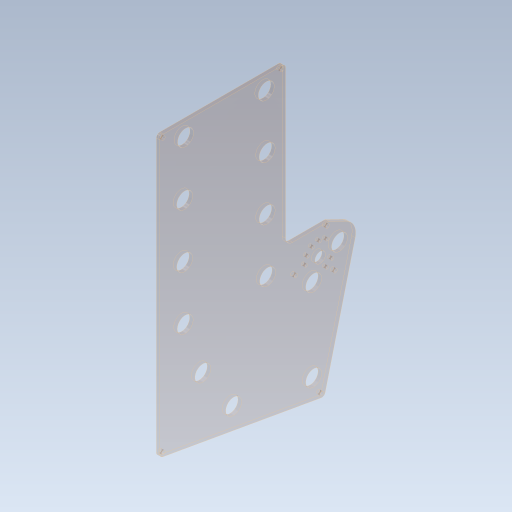
# Autodesk Inventor part: sketchers
Saved by Autodesk Inventor 2024 (Build 280153000, 153)
## iProperties
Created: 2024-07-27
Part Number: sketchers
Material: Polycarbonate, Smoke
Document SubType Name: Modeling
Designer: Oscar
Density: 1.2 g/cm^3
Appearance: Polycarbonate - Smoked
Author: Oscar
Autodesk Inventor part; units mm, degrees
ref_plane "YZ Plane" through (0, 0, 0) normal (1, 0, 0) x (0, 1, 0)
ref_plane "XZ Plane" through (0, 0, 0) normal (0, 1, 0) x (-1, 0, 0)
ref_plane "XY Plane" through (0, 0, 0) normal (0, 0, 1) x (1, 0, 0)
sketch "Sketch1" plane through (0, 0, 0) normal (1, 0, 0) x (0, 1, 0)
  line L0 (95.25, 812.8) -> (44.45, 812.8) construction
  line L1 (44.45, 812.8) -> (44.45, 0) construction
  line L2 (44.45, 0) -> (95.25, 0) construction
  line L3 (95.25, 0) -> (95.25, 812.8) construction
  line L4 (95.25, 0) -> (44.45, 0) construction
  line L5 (44.45, 0) -> (44.45, 25.4) construction
  line L6 (44.45, 25.4) -> (95.25, 25.4) construction
  line L7 (95.25, 25.4) -> (95.25, 0) construction
  circle A0 centre (190.5, 0) radius 50.8 construction
  circle A1 centre (95.25, 279.4) radius 25.4 construction
  circle A2 centre (278.0133, 267.5807) radius 9.525
  circle A3 centre (278.0133, 267.5807) radius 25.4 construction
  circle A4 centre (278.0133, 267.5807) radius 31.75 construction
  circle A5 centre (303.4133, 267.5807) radius 2.4892
  circle A6 centre (300.0104, 280.2807) radius 2.4892
  circle A7 centre (290.7133, 289.5778) radius 2.4892
  circle A8 centre (278.0133, 292.9807) radius 2.4892
  circle A9 centre (265.3133, 289.5778) radius 2.4892 construction
  circle A10 centre (256.0163, 280.2807) radius 2.4892 construction
  circle A11 centre (252.6133, 267.5807) radius 2.4892 construction
  circle A12 centre (256.0163, 254.8807) radius 2.4892
  circle A13 centre (265.3133, 245.5837) radius 2.4892
  circle A14 centre (278.0133, 242.1807) radius 2.4892 construction
  circle A15 centre (290.7133, 245.5837) radius 2.4892 construction
  circle A16 centre (300.0104, 254.8807) radius 2.4892
  circle A17 centre (609.6, 438.15) radius 50.8 construction
  circle A18 centre (278.0133, 267.5807) radius 30.48 construction
  circle A19 centre (587.8333, 365.125) radius 25.4 construction
  circle A20 centre (587.8333, 511.175) radius 25.4 construction
  line L8 (587.8333, 485.775) -> (587.8333, 390.525) construction
  circle A21 centre (490.3356, 512.7625) radius 14.351
  circle A22 centre (392.825, 512.7625) radius 14.351
  circle A23 centre (490.3356, 363.5375) radius 14.351
  line L9 (587.8333, 511.175) -> (490.3356, 512.7625) construction
  line L10 (587.8333, 365.125) -> (490.3356, 363.5375) construction
  circle A24 centre (490.3356, 512.7625) radius 25.4 construction
  circle A25 centre (490.3356, 363.5375) radius 25.4 construction
  line L11 (490.3356, 487.3625) -> (490.3356, 388.9375) construction
  circle A26 centre (392.825, 512.7625) radius 25.4 construction
  circle A27 centre (392.825, 363.5375) radius 25.4 construction
  circle A28 centre (392.825, 363.5375) radius 14.351
  line L12 (490.3356, 512.7625) -> (392.825, 512.7625) construction
  line L13 (490.3356, 363.5375) -> (392.825, 363.5375) construction
  line L14 (392.825, 487.3625) -> (392.825, 388.9375) construction
  circle A29 centre (295.3189, 511.8309) radius 25.4 construction
  circle A30 centre (295.3189, 362.6059) radius 25.4 construction
  circle A31 centre (203.1597, 479.9719) radius 25.4 construction
  circle A32 centre (295.3189, 511.8309) radius 14.351
  circle A33 centre (295.3189, 362.6059) radius 14.351
  circle A34 centre (203.1597, 479.9719) radius 14.351
  line L15 (392.825, 512.7625) -> (295.3189, 511.8309) construction
  line L16 (392.825, 363.5375) -> (295.3189, 362.6059) construction
  line L17 (295.3189, 486.4309) -> (295.3189, 388.0059) construction
  line L18 (295.3189, 511.8309) -> (203.1597, 479.9719) construction
  circle A35 centre (123.1487, 424.2353) radius 25.4 construction
  circle A36 centre (123.1487, 424.2353) radius 14.351
  line L19 (203.1597, 479.9719) -> (123.1487, 424.2353) construction
  circle A37 centre (95.25, 279.4) radius 14.351
  circle A38 centre (407.176, 125.0684) radius 50.8 construction
  line L20 (609.6, 355.6) -> (44.45, 355.6) construction
  line L21 (44.45, 355.6) -> (44.45, 330.2) construction
  line L22 (44.45, 330.2) -> (609.6, 330.2) construction
  line L23 (609.6, 330.2) -> (609.6, 355.6) construction
  line L24 (95.25, 241.3) -> (44.45, 241.3) construction
  line L25 (44.45, 241.3) -> (44.45, 215.9) construction
  line L26 (44.45, 215.9) -> (95.25, 215.9) construction
  line L27 (95.25, 215.9) -> (95.25, 241.3) construction
  circle A39 centre (244.475, 279.4) radius 25.4 construction
  circle A40 centre (244.475, 279.4) radius 14.351
  line L28 (218.8463, 459.9947) -> (279.6322, 382.5831) construction
  circle A41 centre (278.0133, 267.5807) radius 8.89 construction
  circle A42 centre (284.5531, 232.6273) radius 26.67 construction
  circle A43 centre (244.475, 279.4) radius 26.67 construction
  circle A44 centre (284.5531, 232.6273) radius 14.351
  circle A45 centre (587.8333, 511.175) radius 14.351
  circle A46 centre (587.8333, 365.125) radius 14.351
  line L29 (44.45, 623.1841) -> (44.45, 648.5841) construction
  line L30 (95.25, 647.7) -> (609.6, 647.7) construction
  line L31 (609.6, 647.7) -> (609.6, 622.3) construction
  line L32 (609.6, 622.3) -> (95.25, 622.3) construction
  line L33 (95.25, 622.3) -> (95.25, 647.7) construction
  circle A47 centre (606.8833, 551.3359) radius 3.2639
  circle A48 centre (606.8833, 551.3359) radius 6.35 construction
  circle A49 centre (606.8833, 336.55) radius 3.2639
  circle A50 centre (606.8833, 336.55) radius 6.35 construction
  circle A51 centre (114.3, 551.3359) radius 3.2639
  circle A52 centre (114.3, 551.3359) radius 6.35 construction
  line L34 (598.719, 534.1241) -> (604.1619, 545.5987) construction
  line L35 (613.2333, 551.3359) -> (613.2333, 511.175)
  line L36 (613.2333, 365.125) -> (613.2333, 336.55)
  line L37 (613.2333, 511.175) -> (613.2333, 365.125)
  circle A53 centre (63.5, 264.8503) radius 3.2639
  circle A54 centre (63.5, 264.8503) radius 6.35 construction
  line L38 (339.48, 330.2) -> (606.8833, 330.2)
  line L39 (313.4556, 344.8233) -> (322.5239, 335.932) construction
  circle A55 centre (284.5531, 232.6273) radius 29.21 construction
  circle A56 centre (244.475, 279.4) radius 29.21 construction
  arc A57 (606.8833, 330.2) -> (613.2333, 336.55) centre (606.8833, 336.55) ccw
  line L40 (72.1591, 268.8184) -> (69.2727, 267.4957) construction
  line L41 (609.6, 342.9) -> (44.45, 342.9) construction
  circle A58 centre (284.5531, 232.6273) radius 19.05 construction
  line L42 (263.4811, 257.2191) -> (265.547, 254.8082) construction
  circle A59 centre (320.43, 254.2906) radius 3.2639
  circle A60 centre (271.3806, 311.5331) radius 3.2639
  circle A61 centre (243.2709, 239.8541) radius 3.2639
  line L43 (95.25, 558.8) -> (44.45, 558.8) construction
  line L44 (44.45, 558.8) -> (44.45, 533.4) construction
  line L45 (44.45, 533.4) -> (95.25, 533.4) construction
  line L46 (95.25, 533.4) -> (95.25, 558.8) construction
  line L47 (114.3, 557.6859) -> (606.8833, 557.6859)
  line L48 (108.0475, 552.4446) -> (57.2475, 265.959)
  line L49 (277.4039, 204.3057) -> (61.9458, 258.6935)
  circle A62 centre (320.43, 254.2906) radius 6.35 construction
  circle A63 centre (271.3806, 311.5331) radius 6.35 construction
  circle A64 centre (243.2709, 239.8541) radius 6.35 construction
  arc A65 (114.3, 557.6859) -> (108.0475, 552.4446) centre (114.3, 551.3359) ccw
  arc A66 (57.2475, 265.959) -> (61.9458, 258.6935) centre (63.5, 264.8503) ccw
  line L50 (314.3705, 256.1892) -> (308.3109, 258.0878) construction
  line L51 (314.9941, 251.0083) -> (309.5582, 247.7259) construction
  line L52 (272.3281, 305.2542) -> (273.2757, 298.9753) construction
  line L53 (267.304, 306.6644) -> (263.2274, 301.7958) construction
  line L54 (249.5258, 238.7591) -> (255.7807, 237.6641) construction
  line L55 (248.2341, 243.815) -> (253.1973, 247.776) construction
  line L56 (326.78, 317.5) -> (326.78, 254.2906)
  arc A67 (339.48, 330.2) -> (326.78, 317.5) centre (339.48, 317.5) ccw
  line L57 (326.1461, 251.5249) -> (310.8471, 219.9051)
  arc A68 (326.1461, 251.5249) -> (326.78, 254.2906) centre (320.43, 254.2906) ccw
  arc A69 (277.4039, 204.3057) -> (310.8471, 219.9051) centre (284.5531, 232.6273) ccw
  arc A70 (613.2333, 551.3359) -> (606.8833, 557.6859) centre (606.8833, 551.3359) ccw
  point P0 (0, 0)
  point P1 (273.7117, 242.0302)
  point P2 (272.9427, 241.0623)
  point P3 (254.5339, 269.1643)
  point P4 (250.4488, 266.3515)
  dimension "d9" = 50.8
  dimension "d14" = 50.8
  dimension "d53" = 50.8
  dimension "d1" = 812.8
  dimension "d2" = 44.45
  dimension "d4" = 25.4
  dimension "d5" = 101.6
  dimension "d6" = 95.25
  dimension "d8" = 50.8
  dimension "d15" = 63.5
  dimension "d21" = 19.05
  dimension "d26" = 360
  dimension "d28" = 4.9784
  dimension "d29" = 438.15
  dimension "d30" = 514.35
  dimension "d36" = 60.96
  dimension "d38" = 50.8
  dimension "d39" = 50.8
  dimension "d41" = 95.25
  dimension "d45" = 28.702
  dimension "d47" = 97.5106
  dimension "d48" = 98.425
  dimension "d56" = 25.4
  dimension "d73" = 50.8
  dimension "d74" = 25.4
  dimension "d75" = 215.9
  dimension "d78" = 279.4
  dimension "d80" = 149.225
  dimension "d81" = 97.5106
  dimension "d82" = 147.4978
  dimension "d83" = 17.78
  dimension "d85" = 53.34
  dimension "d92" = 330.2
  dimension "d100" = 514.35
  dimension "d107" = 25.4
  dimension "d108" = 514.35
  dimension "d109" = 266.7
  dimension "d110" = 12.7
  dimension "d115" = 6.5278
  dimension "d116" = 12.7
  dimension "d122" = 2.54
  dimension "d123" = 2.54
  dimension "d128" = 3.175
  dimension "d133" = 38.1
  dimension "d134" = 3.175
  dimension "d135" = 194.9958
  dimension "d136" = 6.5278
  dimension "d137" = 25.4
  dimension "d138" = 533.4
  dimension "d139" = 19.05
  dimension "d140" = 19.05
  dimension "d141" = 12.7
  dimension "d142" = 6.35
  dimension "d143" = 12.7
  constraints: 114 end point, 63 centre point, 51 point on circle, 32 point on line, 27 coincident, 25 tangent, 24 equal radius, 15 equal length, 11 parallel, 9 horizontal, 7 vertical alignment, 6 horizontal alignment, 6 perpendicular, 4 concentric, 4 vertical, 2 midpoint, 53 other
  measures "d1" distance of L1.end L0.end
  measures "d2" distance from line of point (0, 0) L1
  measures "d4" distance of L4.end L5.end
  measures "d5" diameter of A0
  measures "d15" diameter of A4
  measures "d21" diameter of A2
  measures "d28" diameter of A16
  measures "d29" distance from line of L2 point (609.6, 438.15)
  measures "d36" diameter of A18
  measures "d38" diameter of A19
  measures "d39" diameter of A20
  measures "d41" distance of L8.start L8.end
  measures "d45" diameter of A21
  measures "d47" distance of L9.start L9.end
  measures "d48" distance of L11.start L11.end
  measures "d56" distance of L22.end L20.start
  measures "d73" distance of L26.end L25.end
  measures "d74" distance of L25.end L24.end
  measures "d75" distance between parallel lines of L2 L26
  measures "d78" distance from line of L2 point (95.25, 279.4)
  measures "d80" distance of point (95.25, 279.4) A39.centre
  measures "d81" distance of A39.centre A30.centre
  measures "d82" distance of point (95.25, 279.4) A35.centre
  measures "d83" diameter of A41
  measures "d85" diameter of A42
  measures "d92" distance between parallel lines of L2 L22
  measures "d107" distance between parallel lines of L32 L30
  measures "d108" distance of L31.end L32.end
  measures "d109" distance between parallel lines of L20 L32
  measures "d110" distance of L34.start L34.end
  measures "d115" diameter of A47
  measures "d116" diameter of A48
  measures "d122" radial gap between concentric circles of A42 A55
  measures "d123" radial gap between concentric circles of A43 A56
  measures "d128" distance of L40.start L40.end
  measures "d133" diameter of A58
  measures "d134" distance of L42.start L42.end
  measures "d135" distance of A37.centre A44.centre
  measures "d136" diameter of A61
  measures "d137" distance between parallel lines of L43 L45
  measures "d138" distance between parallel lines of L2 L45
  measures "d140" distance from line of L1 A53.centre
  measures "d141" diameter of A64
  measures "d142" distance of L51.start L51.end
  measures "d143" radius of A67
extrude "Extrusion2" add sketch "Sketch1" along normal blind 6.35
body "Solid2"
